Autodesk Inventor part; units mm, degrees
(part 2 of 3)
  line L954 (9.5722, 12.2732) -> (9.481, 12.2224)
  line L955 (9.481, 12.2224) -> (9.3887, 12.173)
  line L956 (9.3887, 12.173) -> (9.2008, 12.0779)
  line L957 (9.2008, 12.0779) -> (8.8135, 11.9014)
  line L958 (8.8135, 11.9014) -> (8.4127, 11.7415)
  line L959 (8.4127, 11.7415) -> (7.9999, 11.5967)
  line L960 (7.9999, 11.5967) -> (7.5762, 11.4663)
  line L961 (7.5762, 11.4663) -> (7.1423, 11.3497)
  line L962 (7.1423, 11.3497) -> (6.777, 11.8009)
  line L963 (6.777, 11.8009) -> (6.9813, 12.201)
  line L964 (6.9813, 12.201) -> (7.1969, 12.5884)
  line L965 (7.1969, 12.5884) -> (7.4243, 12.9621)
  line L966 (7.4243, 12.9621) -> (7.6641, 13.3208)
  line L967 (7.6641, 13.3208) -> (7.9172, 13.663)
  line L968 (7.9172, 13.663) -> (8.0493, 13.827)
  line L969 (8.0493, 13.827) -> (8.1169, 13.907)
  line L970 (8.1169, 13.907) -> (8.1855, 13.9856)
  line L971 (8.1855, 13.9856) -> (7.7098, 14.6404)
  line L972 (7.7098, 14.6404) -> (7.6138, 14.5994)
  line L973 (7.6138, 14.5994) -> (7.5168, 14.5599)
  line L974 (7.5168, 14.5599) -> (7.32, 14.4849)
  line L975 (7.32, 14.4849) -> (6.9164, 14.3499)
  line L976 (6.9164, 14.3499) -> (6.5011, 14.2327)
  line L977 (6.5011, 14.2327) -> (6.0755, 14.1319)
  line L978 (6.0755, 14.1319) -> (5.6404, 14.0465)
  line L979 (5.6404, 14.0465) -> (5.1967, 13.9759)
  line L980 (5.1967, 13.9759) -> (4.8805, 14.4628)
  line L981 (4.8805, 14.4628) -> (5.1255, 14.8394)
  line L982 (5.1255, 14.8394) -> (5.3805, 15.2021)
  line L983 (5.3805, 15.2021) -> (5.6457, 15.55)
  line L984 (5.6457, 15.55) -> (5.9217, 15.8817)
  line L985 (5.9217, 15.8817) -> (6.2092, 16.1955)
  line L986 (6.2092, 16.1955) -> (6.3577, 16.3448)
  line L987 (6.3577, 16.3448) -> (6.4333, 16.4173)
  line L988 (6.4333, 16.4173) -> (6.5097, 16.4883)
  line L989 (6.5097, 16.4883) -> (6.1051, 17.1892)
  line L990 (6.1051, 17.1892) -> (6.0053, 17.1585)
  line L991 (6.0053, 17.1585) -> (5.9047, 17.1293)
  line L992 (5.9047, 17.1293) -> (5.7012, 17.0754)
  line L993 (5.7012, 17.0754) -> (5.2857, 16.9833)
  line L994 (5.2857, 16.9833) -> (4.8604, 16.9101)
  line L995 (4.8604, 16.9101) -> (4.4265, 16.8544)
  line L996 (4.4265, 16.8544) -> (3.9849, 16.8149)
  line L997 (3.9849, 16.8149) -> (3.5363, 16.7911)
  line L998 (3.5363, 16.7911) -> (3.2727, 17.3084)
  line L999 (3.2727, 17.3084) -> (3.5558, 17.6573)
  line L1000 (3.5558, 17.6573) -> (3.8472, 17.9913)
  line L1001 (3.8472, 17.9913) -> (4.1474, 18.3096)
  line L1002 (4.1474, 18.3096) -> (4.4565, 18.6106)
  line L1003 (4.4565, 18.6106) -> (4.7752, 18.8927)
  line L1004 (4.7752, 18.8927) -> (4.9385, 19.0256)
  line L1005 (4.9385, 19.0256) -> (5.0212, 19.0899)
  line L1006 (5.0212, 19.0899) -> (5.1047, 19.1525)
  line L1007 (5.1047, 19.1525) -> (4.7756, 19.8919)
  line L1008 (4.7756, 19.8919) -> (4.6731, 19.8717)
  line L1009 (4.6731, 19.8717) -> (4.5701, 19.8532)
  line L1010 (4.5701, 19.8532) -> (4.362, 19.8208)
  line L1011 (4.362, 19.8208) -> (3.9391, 19.7727)
  line L1012 (3.9391, 19.7727) -> (3.5085, 19.7444)
  line L1013 (3.5085, 19.7444) -> (3.0712, 19.7343)
  line L1014 (3.0712, 19.7343) -> (2.6279, 19.7412)
  line L1015 (2.6279, 19.7412) -> (2.1792, 19.7644)
  line L1016 (2.1792, 19.7644) -> (1.9712, 20.3064)
  line L1017 (1.9712, 20.3064) -> (2.2891, 20.6238)
  line L1018 (2.2891, 20.6238) -> (2.6139, 20.9256)
  line L1019 (2.6139, 20.9256) -> (2.9457, 21.2107)
  line L1020 (2.9457, 21.2107) -> (3.2846, 21.4778)
  line L1021 (3.2846, 21.4778) -> (3.631, 21.725)
  line L1022 (3.631, 21.725) -> (3.8074, 21.8401)
  line L1023 (3.8074, 21.8401) -> (3.8963, 21.8954)
  line L1024 (3.8963, 21.8954) -> (3.9859, 21.949)
  line L1025 (3.9859, 21.949) -> (3.7358, 22.7186)
  line L1026 (3.7358, 22.7186) -> (3.6319, 22.7093)
  line L1027 (3.6319, 22.7093) -> (3.5274, 22.7017)
  line L1028 (3.5274, 22.7017) -> (3.3171, 22.6913)
  line L1029 (3.3171, 22.6913) -> (2.8915, 22.6876)
  line L1030 (2.8915, 22.6876) -> (2.4603, 22.7045)
  line L1031 (2.4603, 22.7045) -> (2.0243, 22.7401)
  line L1032 (2.0243, 22.7401) -> (1.5842, 22.7933)
  line L1033 (1.5842, 22.7933) -> (1.1404, 22.8633)
  line L1034 (1.1404, 22.8633) -> (0.9901, 23.4241)
  line L1035 (0.9901, 23.4241) -> (1.3395, 23.7065)
  line L1036 (1.3395, 23.7065) -> (1.6941, 23.9727)
  line L1037 (1.6941, 23.9727) -> (2.0538, 24.2216)
  line L1038 (2.0538, 24.2216) -> (2.4188, 24.4518)
  line L1039 (2.4188, 24.4518) -> (2.7892, 24.6613)
  line L1040 (2.7892, 24.6613) -> (2.9766, 24.7575)
  line L1041 (2.9766, 24.7575) -> (3.0708, 24.8031)
  line L1042 (3.0708, 24.8031) -> (3.1655, 24.847)
  line L1043 (3.1655, 24.847) -> (2.9973, 25.6386)
  line L1044 (2.9973, 25.6386) -> (2.8929, 25.6402)
  line L1045 (2.8929, 25.6402) -> (2.7882, 25.6436)
  line L1046 (2.7882, 25.6436) -> (2.5779, 25.6552)
  line L1047 (2.5779, 25.6552) -> (2.1543, 25.696)
  line L1048 (2.1543, 25.696) -> (1.7273, 25.7578)
  line L1049 (1.7273, 25.7578) -> (1.2974, 25.8389)
  line L1050 (1.2974, 25.8389) -> (0.8652, 25.9378)
  line L1051 (0.8652, 25.9378) -> (0.4312, 26.0538)
  line L1052 (0.4312, 26.0538) -> (0.3404, 26.6272)
  line L1053 (0.3404, 26.6272) -> (0.7173, 26.8716)
  line L1054 (0.7173, 26.8716) -> (1.0978, 27.0992)
  line L1055 (1.0978, 27.0992) -> (1.4816, 27.3091)
  line L1056 (1.4816, 27.3091) -> (1.8686, 27.4999)
  line L1057 (1.8686, 27.4999) -> (2.2589, 27.6697)
  line L1058 (2.2589, 27.6697) -> (2.4553, 27.7456)
  line L1059 (2.4553, 27.7456) -> (2.5538, 27.7812)
  line L1060 (2.5538, 27.7812) -> (2.6526, 27.8149)
  line L1061 (2.6526, 27.8149) -> (2.568, 28.6198)
  line L1062 (2.568, 28.6198) -> (2.4644, 28.6323)
  line L1063 (2.4644, 28.6323) -> (2.3606, 28.6466)
  line L1064 (2.3606, 28.6466) -> (2.1527, 28.6801)
  line L1065 (2.1527, 28.6801) -> (1.7356, 28.765)
  line L1066 (1.7356, 28.765) -> (1.3174, 28.8711)
  line L1067 (1.3174, 28.8711) -> (0.8983, 28.9967)
  line L1068 (0.8983, 28.9967) -> (0.4789, 29.1403)
  line L1069 (0.4789, 29.1403) -> (0.0593, 29.3009)
  line L1070 (0.0593, 29.3009) -> (0.029, 29.8807)
  line L1071 (0.029, 29.8807) -> (0.4294, 30.0843)
  line L1072 (0.4294, 30.0843) -> (0.8316, 30.2709)
  line L1073 (0.8316, 30.2709) -> (1.2352, 30.4396)
  line L1074 (1.2352, 30.4396) -> (1.64, 30.5889)
  line L1075 (1.64, 30.5889) -> (2.0459, 30.7169)
  line L1076 (2.0459, 30.7169) -> (2.2492, 30.772)
  line L1077 (2.2492, 30.772) -> (2.3509, 30.797)
  line L1078 (2.3509, 30.797) -> (2.4527, 30.8203)
  line L1079 (2.4527, 30.8203) -> (2.4527, 31.6296)
  circle A0 centre (31.2249, 31.2249) radius 0.5
  line L1080 (62.4057, 32.859) -> (0.0441, 29.5908) construction
derived "Base_part.ipt"
derived "gear_central_part_30.ipt"
sketch "Sketch9" plane through (0, 0, 0) normal (0, 1, 0) x (-1, 0, 0)
  circle A0 centre (0, 0) radius 15
  arc A1 (4.5, -13.2571) -> (5.5, -12.8744) centre (0, 0) ccw
  line L0 (0, 0) -> (20.2233, 0) construction
  line L1 (0, 0) -> (0, -27.3647) construction
  line L2 (0.2121, 2.4395) -> (2.4395, 0.2121)
  line L3 (2.4395, -0.2121) -> (0.2121, -2.4395)
  line L4 (-0.2121, -2.4395) -> (-2.4395, -0.2121)
  line L5 (-2.4395, 0.2121) -> (-0.2121, 2.4395)
  line L6 (0, 2.6517) -> (0, -2.6517) construction
  line L7 (2.6517, 0) -> (-2.6517, 0) construction
  arc A2 (2.4395, -0.2121) -> (2.4395, 0.2121) centre (2.2274, 0) ccw
  arc A3 (-0.2121, -2.4395) -> (0.2121, -2.4395) centre (0, -2.2274) ccw
  arc A4 (-2.4395, 0.2121) -> (-2.4395, -0.2121) centre (-2.2274, 0) ccw
  arc A5 (0.2121, 2.4395) -> (-0.2121, 2.4395) centre (0, 2.2274) ccw
  line L8 (-3.1466, -0.9192) -> (-0.9192, -3.1466)
  arc A6 (-0.9192, -3.1466) -> (0.9192, -3.1466) centre (0, -2.2274) ccw
  line L9 (0.9192, -3.1466) -> (3.1466, -0.9192)
  arc A7 (3.1466, -0.9192) -> (3.1466, 0.9192) centre (2.2274, 0) ccw
  line L10 (3.1466, 0.9192) -> (0.9192, 3.1466)
  arc A8 (0.9192, 3.1466) -> (-0.9192, 3.1466) centre (0, 2.2274) ccw
  line L11 (-0.9192, 3.1466) -> (-3.1466, 0.9192)
  arc A9 (-3.1466, 0.9192) -> (-3.1466, -0.9192) centre (-2.2274, 0) ccw
  circle A10 centre (10, 0) radius 2.5
  arc A11 (13.4641, -0.5) -> (9.5, -3.4641) centre (10, 0) ccw
  line L12 (3.4274, -0.5) -> (6.5359, -0.5)
  line L13 (3.4274, 0.5) -> (6.5359, 0.5)
  line L14 (13.9911, 0.5) -> (13.4641, 0.5)
  line L15 (13.9911, -0.5) -> (13.4641, -0.5)
  line L16 (0, -5) -> (13.0767, -5) construction
  line L17 (0, -4.5) -> (13.2571, -4.5)
  line L18 (0, -5.5) -> (12.8744, -5.5)
  line L19 (5, 0) -> (5, -13.0767) construction
  line L20 (5.5, 12.8744) -> (5.5, -12.8744)
  line L21 (4.5, 13.2571) -> (4.5, -13.2571)
  arc A12 (0, -14) -> (4.5, -13.2571) centre (0, 0) ccw
  arc A13 (5.5, -12.8744) -> (12.8744, -5.5) centre (0, 0) ccw
  arc A14 (12.8744, -5.5) -> (13.2571, -4.5) centre (0, 0) ccw
  arc A15 (13.2571, -4.5) -> (13.9911, -0.5) centre (0, 0) ccw
  arc A16 (13.9911, -0.5) -> (13.9911, 0.5) centre (0, 0) ccw
  arc A17 (13.9911, 0.5) -> (5.5, 12.8744) centre (0, 0) ccw
  line L22 (0.5, -4.5) -> (0.5, -5.5)
  line L23 (10, 0) -> (10, -4.5) construction
  line L24 (10.5, -3.4641) -> (10.5, -4.5)
  line L25 (9.5, -3.4641) -> (9.5, -4.5)
  arc A18 (10.5, -3.4641) -> (13.4641, -0.5) centre (10, 0) ccw
  arc A19 (9.5, -3.4641) -> (10.5, -3.4641) centre (10, 0) ccw
  arc A20 (10.5, 3.4641) -> (9.5, 3.4641) centre (10, 0) ccw
  line L26 (0, -4.5) -> (0, -5.5)
  arc A21 (4.5, 13.2571) -> (0, -14) centre (0, 0) ccw
  arc A22 (5.5, 12.8744) -> (4.5, 13.2571) centre (0, 0) ccw
  line L27 (0, 4.5) -> (0, 5.5)
  line L28 (9.5, 3.4641) -> (9.5, 4.5)
  arc A23 (10.5, 3.4641) -> (9.5, 3.4641) centre (10, 0) ccw
  line L29 (0.5, 4.5) -> (0.5, 5.5)
  line L30 (0, 4.5) -> (13.2571, 4.5)
  line L31 (0, 5) -> (13.0767, 5) construction
  line L32 (0, 5.5) -> (12.8744, 5.5)
  arc A24 (13.2571, 4.5) -> (12.8744, 5.5) centre (0, 0) ccw
  line L33 (10.5, 3.4641) -> (10.5, 4.5)
  arc A25 (2.4395, -0.2121) -> (2.4395, 0.2121) centre (2.2274, 0) ccw
  line L34 (0.2121, 2.4395) -> (2.4395, 0.2121)
  line L35 (0.9192, -3.1466) -> (3.1466, -0.9192)
  arc A26 (0.2121, 2.4395) -> (-0.2121, 2.4395) centre (0, 2.2274) ccw
  line L36 (2.4395, -0.2121) -> (0.2121, -2.4395)
  line L37 (0, 2.6517) -> (0, -2.6517) construction
  line L38 (-2.4395, 0.2121) -> (-0.2121, 2.4395)
  line L39 (-2.6517, 0) -> (2.6517, 0) construction
  arc A27 (-0.2121, -2.4395) -> (0.2121, -2.4395) centre (0, -2.2274) ccw
  line L40 (-0.2121, -2.4395) -> (-2.4395, -0.2121)
  arc A28 (3.1466, -0.9192) -> (3.1466, 0.9192) centre (2.2274, 0) ccw
  line L41 (3.1466, 0.9192) -> (0.9192, 3.1466)
  line L42 (4.5, 0.5) -> (5.5, 0.5)
  line L43 (4.5, 0) -> (5.5, 0)
  line L44 (-13.2571, 4.5) -> (13.2571, 4.5)
  line L45 (0, 5) -> (13.0767, 5) construction
  arc A29 (14, 0) -> (13.2571, 4.5) centre (0, 0) ccw
  arc A30 (-0.9192, -3.1466) -> (0.9192, -3.1466) centre (0, -2.2274) ccw
  line L46 (-3.1466, -0.9192) -> (-0.9192, -3.1466)
  arc A31 (-12.8744, 5.5) -> (-13.2571, 4.5) centre (0, 0) ccw
  circle A32 centre (0, 10) radius 2.5
  arc A33 (0.5, 13.4641) -> (3.4641, 9.5) centre (0, 10) ccw
  line L47 (0.5, 3.4274) -> (0.5, 6.5359)
  line L48 (-0.5, 3.4274) -> (-0.5, 6.5359)
  arc A34 (3.4641, 10.5) -> (0.5, 13.4641) centre (0, 10) ccw
  line L49 (0, 10) -> (4.5, 10) construction
  line L50 (0.5, 13.9911) -> (0.5, 13.4641)
  arc A35 (4.5, 13.2571) -> (0.5, 13.9911) centre (0, 0) ccw
  line L51 (-12.8744, 5.5) -> (12.8744, 5.5)
  arc A36 (0.5, 13.9911) -> (-0.5, 13.9911) centre (0, 0) ccw
  line L52 (-0.5, 13.9911) -> (-0.5, 13.4641)
  arc A37 (13.2571, 4.5) -> (12.8744, 5.5) centre (0, 0) ccw
  arc A38 (3.4641, 9.5) -> (3.4641, 10.5) centre (0, 10) ccw
  line L53 (3.4641, 9.5) -> (4.5, 9.5)
  line L54 (3.4641, 10.5) -> (4.5, 10.5)
  arc A39 (5.5, 12.8744) -> (4.5, 13.2571) centre (0, 0) ccw
  line L55 (4.5, 0) -> (4.5, 13.2571)
  line L56 (5, 0) -> (5, 13.0767) construction
  line L57 (5.5, 0) -> (5.5, 12.8744)
  arc A40 (12.8744, 5.5) -> (5.5, 12.8744) centre (0, 0) ccw
  line L58 (-0.9192, 3.1466) -> (-3.1466, 0.9192)
  arc A41 (-3.4641, 10.5) -> (-3.4641, 9.5) centre (0, 10) ccw
  arc A42 (-3.4641, 10.5) -> (-3.4641, 9.5) centre (0, 10) ccw
  line L59 (-3.4641, 10.5) -> (-4.5, 10.5)
  line L60 (-4.5, 0) -> (-4.5, 13.2571)
  line L61 (-5, 0) -> (-5, 13.0767) construction
  line L62 (-5.5, 0) -> (-5.5, 12.8744)
  arc A43 (-4.5, 13.2571) -> (-5.5, 12.8744) centre (0, 0) ccw
  arc A44 (-0.5, 13.9911) -> (-12.8744, 5.5) centre (0, 0) ccw
  line L63 (-3.4641, 9.5) -> (-4.5, 9.5)
  line L64 (-4.5, 0.5) -> (-5.5, 0.5)
  line L65 (-4.5, 0) -> (-5.5, 0)
  arc A45 (-2.4395, 0.2121) -> (-2.4395, -0.2121) centre (-2.2274, 0) ccw
  arc A46 (-3.1466, 0.9192) -> (-3.1466, -0.9192) centre (-2.2274, 0) ccw
  arc A47 (0.9192, 3.1466) -> (-0.9192, 3.1466) centre (0, 2.2274) ccw
  arc A48 (0.2121, 2.4395) -> (-0.2121, 2.4395) centre (0, 2.2274) ccw
  line L66 (-2.4395, 0.2121) -> (-0.2121, 2.4395)
  line L67 (3.1466, 0.9192) -> (0.9192, 3.1466)
  arc A49 (-2.4395, 0.2121) -> (-2.4395, -0.2121) centre (-2.2274, 0) ccw
  line L68 (0.2121, 2.4395) -> (2.4395, 0.2121)
  line L69 (-2.6517, 0) -> (2.6517, 0) construction
  line L70 (-0.2121, -2.4395) -> (-2.4395, -0.2121)
  line L71 (0, -2.6517) -> (0, 2.6517) construction
  arc A50 (2.4395, -0.2121) -> (2.4395, 0.2121) centre (2.2274, 0) ccw
  line L72 (2.4395, -0.2121) -> (0.2121, -2.4395)
  arc A51 (0.9192, 3.1466) -> (-0.9192, 3.1466) centre (0, 2.2274) ccw
  line L73 (-0.9192, 3.1466) -> (-3.1466, 0.9192)
  line L74 (-0.5, 4.5) -> (-0.5, 5.5)
  line L75 (0, 4.5) -> (0, 5.5)
  line L76 (-4.5, -13.2571) -> (-4.5, 13.2571)
  line L77 (-5, 0) -> (-5, 13.0767) construction
  arc A52 (0, 14) -> (-4.5, 13.2571) centre (0, 0) ccw
  arc A53 (3.1466, -0.9192) -> (3.1466, 0.9192) centre (2.2274, 0) ccw
  line L78 (0.9192, -3.1466) -> (3.1466, -0.9192)
  arc A54 (-5.5, -12.8744) -> (-4.5, -13.2571) centre (0, 0) ccw
  circle A55 centre (-10, 0) radius 2.5
  arc A56 (-13.4641, 0.5) -> (-9.5, 3.4641) centre (-10, 0) ccw
  line L79 (-3.4274, 0.5) -> (-6.5359, 0.5)
  line L80 (-3.4274, -0.5) -> (-6.5359, -0.5)
  arc A57 (-10.5, 3.4641) -> (-13.4641, 0.5) centre (-10, 0) ccw
  line L81 (-10, 0) -> (-10, 4.5) construction
  line L82 (-13.9911, 0.5) -> (-13.4641, 0.5)
  arc A58 (-13.2571, 4.5) -> (-13.9911, 0.5) centre (0, 0) ccw
  line L83 (-5.5, -12.8744) -> (-5.5, 12.8744)
  arc A59 (-13.9911, 0.5) -> (-13.9911, -0.5) centre (0, 0) ccw
  line L84 (-13.9911, -0.5) -> (-13.4641, -0.5)
  arc A60 (-4.5, 13.2571) -> (-5.5, 12.8744) centre (0, 0) ccw
  arc A61 (-9.5, 3.4641) -> (-10.5, 3.4641) centre (-10, 0) ccw
  line L85 (-9.5, 3.4641) -> (-9.5, 4.5)
  line L86 (-10.5, 3.4641) -> (-10.5, 4.5)
  arc A62 (-12.8744, 5.5) -> (-13.2571, 4.5) centre (0, 0) ccw
  line L87 (0, 4.5) -> (-13.2571, 4.5)
  line L88 (0, 5) -> (-13.0767, 5) construction
  line L89 (0, 5.5) -> (-12.8744, 5.5)
  arc A63 (-5.5, 12.8744) -> (-12.8744, 5.5) centre (0, 0) ccw
  line L90 (-3.1466, -0.9192) -> (-0.9192, -3.1466)
  arc A64 (-10.5, -3.4641) -> (-9.5, -3.4641) centre (-10, 0) ccw
  arc A65 (-10.5, -3.4641) -> (-9.5, -3.4641) centre (-10, 0) ccw
  line L91 (-10.5, -3.4641) -> (-10.5, -4.5)
  line L92 (0, -4.5) -> (-13.2571, -4.5)
  line L93 (0, -5) -> (-13.0767, -5) construction
  line L94 (0, -5.5) -> (-12.8744, -5.5)
  arc A66 (-13.2571, -4.5) -> (-12.8744, -5.5) centre (0, 0) ccw
  arc A67 (-13.9911, -0.5) -> (-5.5, -12.8744) centre (0, 0) ccw
  line L95 (-9.5, -3.4641) -> (-9.5, -4.5)
  line L96 (-0.5, -4.5) -> (-0.5, -5.5)
  line L97 (0, -4.5) -> (0, -5.5)
  arc A68 (-0.2121, -2.4395) -> (0.2121, -2.4395) centre (0, -2.2274) ccw
  arc A69 (-0.9192, -3.1466) -> (0.9192, -3.1466) centre (0, -2.2274) ccw
  arc A70 (-3.1466, 0.9192) -> (-3.1466, -0.9192) centre (-2.2274, 0) ccw
  arc A71 (-2.4395, 0.2121) -> (-2.4395, -0.2121) centre (-2.2274, 0) ccw
  line L98 (-0.2121, -2.4395) -> (-2.4395, -0.2121)
  line L99 (-0.9192, 3.1466) -> (-3.1466, 0.9192)
  arc A72 (-0.2121, -2.4395) -> (0.2121, -2.4395) centre (0, -2.2274) ccw
  line L100 (-2.4395, 0.2121) -> (-0.2121, 2.4395)
  line L101 (0, -2.6517) -> (0, 2.6517) construction
  line L102 (2.4395, -0.2121) -> (0.2121, -2.4395)
  line L103 (2.6517, 0) -> (-2.6517, 0) construction
  arc A73 (0.2121, 2.4395) -> (-0.2121, 2.4395) centre (0, 2.2274) ccw
  line L104 (0.2121, 2.4395) -> (2.4395, 0.2121)
  arc A74 (-3.1466, 0.9192) -> (-3.1466, -0.9192) centre (-2.2274, 0) ccw
  line L105 (-3.1466, -0.9192) -> (-0.9192, -3.1466)
  line L106 (-4.5, -0.5) -> (-5.5, -0.5)
  line L107 (-4.5, 0) -> (-5.5, 0)
  line L108 (13.2571, -4.5) -> (-13.2571, -4.5)
  line L109 (0, -5) -> (-13.0767, -5) construction
  arc A75 (-14, 0) -> (-13.2571, -4.5) centre (0, 0) ccw
  arc A76 (0.9192, 3.1466) -> (-0.9192, 3.1466) centre (0, 2.2274) ccw
  line L110 (3.1466, 0.9192) -> (0.9192, 3.1466)
  arc A77 (12.8744, -5.5) -> (13.2571, -4.5) centre (0, 0) ccw
  circle A78 centre (0, -10) radius 2.5
  arc A79 (-0.5, -13.4641) -> (-3.4641, -9.5) centre (0, -10) ccw
  line L111 (-0.5, -3.4274) -> (-0.5, -6.5359)
  line L112 (0.5, -3.4274) -> (0.5, -6.5359)
  arc A80 (-3.4641, -10.5) -> (-0.5, -13.4641) centre (0, -10) ccw
  line L113 (0, -10) -> (-4.5, -10) construction
  line L114 (-0.5, -13.9911) -> (-0.5, -13.4641)
  arc A81 (-4.5, -13.2571) -> (-0.5, -13.9911) centre (0, 0) ccw
  line L115 (12.8744, -5.5) -> (-12.8744, -5.5)
  arc A82 (-0.5, -13.9911) -> (0.5, -13.9911) centre (0, 0) ccw
  line L116 (0.5, -13.9911) -> (0.5, -13.4641)
  arc A83 (-13.2571, -4.5) -> (-12.8744, -5.5) centre (0, 0) ccw
  arc A84 (-3.4641, -9.5) -> (-3.4641, -10.5) centre (0, -10) ccw
  line L117 (-3.4641, -9.5) -> (-4.5, -9.5)
  line L118 (-3.4641, -10.5) -> (-4.5, -10.5)
  arc A85 (-5.5, -12.8744) -> (-4.5, -13.2571) centre (0, 0) ccw
  line L119 (-4.5, 0) -> (-4.5, -13.2571)
  line L120 (-5, 0) -> (-5, -13.0767) construction
  line L121 (-5.5, 0) -> (-5.5, -12.8744)
  arc A86 (-12.8744, -5.5) -> (-5.5, -12.8744) centre (0, 0) ccw
  line L122 (0.9192, -3.1466) -> (3.1466, -0.9192)
  arc A87 (3.4641, -10.5) -> (3.4641, -9.5) centre (0, -10) ccw
  arc A88 (3.4641, -10.5) -> (3.4641, -9.5) centre (0, -10) ccw
  line L123 (3.4641, -10.5) -> (4.5, -10.5)
  line L124 (4.5, 0) -> (4.5, -13.2571)
  line L125 (5, 0) -> (5, -13.0767) construction
  line L126 (5.5, 0) -> (5.5, -12.8744)
  arc A89 (4.5, -13.2571) -> (5.5, -12.8744) centre (0, 0) ccw
  arc A90 (0.5, -13.9911) -> (12.8744, -5.5) centre (0, 0) ccw
  line L127 (3.4641, -9.5) -> (4.5, -9.5)
  line L128 (4.5, -0.5) -> (5.5, -0.5)
  line L129 (4.5, 0) -> (5.5, 0)
  arc A91 (2.4395, -0.2121) -> (2.4395, 0.2121) centre (2.2274, 0) ccw
  arc A92 (3.1466, -0.9192) -> (3.1466, 0.9192) centre (2.2274, 0) ccw
  arc A93 (-0.9192, -3.1466) -> (0.9192, -3.1466) centre (0, -2.2274) ccw
  point P0 (0, 2.2274)
  point P1 (10, 4.5)
  point P2 (-4.5, 10)
  point P3 (-2.2274, 0)
  point P4 (-10, -4.5)
  point P5 (0, -2.2274)
  point P6 (4.5, -10)
  point P7 (2.2274, 0)
sketch "Sketch7" plane through (0, 0, 0) normal (0, 1, 0) x (-1, 0, 0)
  line L0 (0, 31.2236) -> (0, -31.2236) construction
  arc A0 (4.5, 27.4052) -> (-4.5, 27.4052) centre (0, 0) ccw
  line L1 (5.5, 13.9553) -> (5.5, 27.2222)
  line L2 (4.5, 14.3091) -> (4.5, 27.4052)
  line L3 (5.5, 0) -> (5.5, 12.8744) projected
  line L4 (4.5, 0) -> (4.5, 13.2571) projected
  line L5 (-4.5, 0) -> (-4.5, 13.2571) projected
  line L6 (-5.5, -12.8744) -> (-5.5, 12.8744) projected
  circle A1 centre (0, 0) radius 15 projected
  line L7 (-4.5, 14.3091) -> (-4.5, 27.4052)
  line L8 (-5.5, 13.9553) -> (-5.5, 27.2222)
  arc A2 (5.5, 27.2222) -> (4.5, 27.4052) centre (0, 0) ccw
  arc A3 (-5.5, 27.2222) -> (5.5, 27.2222) centre (0, 0) ccw
  arc A4 (-4.5, 27.4052) -> (-5.5, 27.2222) centre (0, 0) ccw
  arc A5 (5.5, 13.9553) -> (4.5, 14.3091) centre (0, 0) ccw
  arc A6 (-4.5, 14.3091) -> (-5.5, 13.9553) centre (0, 0) ccw
  arc A7 (-14.3091, -4.5) -> (-13.9553, -5.5) centre (0, 0) ccw
  arc A8 (-13.9553, 5.5) -> (-14.3091, 4.5) centre (0, 0) ccw
  line L9 (-13.9553, 5.5) -> (-27.2222, 5.5)
  line L10 (-14.3091, 4.5) -> (-27.4052, 4.5)
  arc A9 (-27.2222, 5.5) -> (-27.4052, 4.5) centre (0, 0) ccw
  line L11 (-14.3091, -4.5) -> (-27.4052, -4.5)
  line L12 (-13.9553, -5.5) -> (-27.2222, -5.5)
  arc A10 (-27.4052, -4.5) -> (-27.2222, -5.5) centre (0, 0) ccw
  arc A11 (4.5, -14.3091) -> (5.5, -13.9553) centre (0, 0) ccw
  arc A12 (-5.5, -13.9553) -> (-4.5, -14.3091) centre (0, 0) ccw
  line L13 (-5.5, -13.9553) -> (-5.5, -27.2222)
  line L14 (-4.5, -14.3091) -> (-4.5, -27.4052)
  arc A13 (-5.5, -27.2222) -> (-4.5, -27.4052) centre (0, 0) ccw
  line L15 (4.5, -14.3091) -> (4.5, -27.4052)
  line L16 (5.5, -13.9553) -> (5.5, -27.2222)
  arc A14 (4.5, -27.4052) -> (5.5, -27.2222) centre (0, 0) ccw
  arc A15 (14.3091, 4.5) -> (13.9553, 5.5) centre (0, 0) ccw
  arc A16 (13.9553, -5.5) -> (14.3091, -4.5) centre (0, 0) ccw
  line L17 (13.9553, -5.5) -> (27.2222, -5.5)
  line L18 (14.3091, -4.5) -> (27.4052, -4.5)
  arc A17 (27.2222, -5.5) -> (27.4052, -4.5) centre (0, 0) ccw
  line L19 (14.3091, 4.5) -> (27.4052, 4.5)
  line L20 (13.9553, 5.5) -> (27.2222, 5.5)
  arc A18 (27.4052, 4.5) -> (27.2222, 5.5) centre (0, 0) ccw
  arc A19 (14.7224, 8.5) -> (8.5, 14.7224) centre (0, 0) ccw
  line L21 (16.4545, 7.5) -> (21.7915, 7.5)
  line L22 (7.5, 16.4545) -> (7.5, 21.7915)
  arc A20 (23.6249, 10.2993) -> (10.2993, 23.6249) centre (0, 0) ccw
  arc A21 (21.7915, 7.5) -> (23.6249, 10.2993) centre (21.7915, 9.5) ccw
  arc A22 (14.7224, 8.5) -> (16.4545, 7.5) centre (16.4545, 9.5) ccw
  arc A23 (7.5, 16.4545) -> (8.5, 14.7224) centre (9.5, 16.4545) ccw
  arc A24 (10.2993, 23.6249) -> (7.5, 21.7915) centre (9.5, 21.7915) ccw
  arc A25 (-16.4545, 7.5) -> (-14.7224, 8.5) centre (-16.4545, 9.5) ccw
  line L23 (-16.4545, 7.5) -> (-21.7915, 7.5)
  arc A26 (-23.6249, 10.2993) -> (-21.7915, 7.5) centre (-21.7915, 9.5) ccw
  arc A27 (-8.5, 14.7224) -> (-14.7224, 8.5) centre (0, 0) ccw
  arc A28 (-10.2993, 23.6249) -> (-23.6249, 10.2993) centre (0, 0) ccw
  arc A29 (-8.5, 14.7224) -> (-7.5, 16.4545) centre (-9.5, 16.4545) ccw
  line L24 (-7.5, 16.4545) -> (-7.5, 21.7915)
  arc A30 (-7.5, 21.7915) -> (-10.2993, 23.6249) centre (-9.5, 21.7915) ccw
  arc A31 (-7.5, -16.4545) -> (-8.5, -14.7224) centre (-9.5, -16.4545) ccw
  line L25 (-7.5, -16.4545) -> (-7.5, -21.7915)
  arc A32 (-10.2993, -23.6249) -> (-7.5, -21.7915) centre (-9.5, -21.7915) ccw
  arc A33 (-14.7224, -8.5) -> (-8.5, -14.7224) centre (0, 0) ccw
  arc A34 (-23.6249, -10.2993) -> (-10.2993, -23.6249) centre (0, 0) ccw
  arc A35 (-14.7224, -8.5) -> (-16.4545, -7.5) centre (-16.4545, -9.5) ccw
  line L26 (-16.4545, -7.5) -> (-21.7915, -7.5)
  arc A36 (-21.7915, -7.5) -> (-23.6249, -10.2993) centre (-21.7915, -9.5) ccw
  arc A37 (16.4545, -7.5) -> (14.7224, -8.5) centre (16.4545, -9.5) ccw
  line L27 (16.4545, -7.5) -> (21.7915, -7.5)
  arc A38 (23.6249, -10.2993) -> (21.7915, -7.5) centre (21.7915, -9.5) ccw
  arc A39 (8.5, -14.7224) -> (14.7224, -8.5) centre (0, 0) ccw
  arc A40 (10.2993, -23.6249) -> (23.6249, -10.2993) centre (0, 0) ccw
  arc A41 (8.5, -14.7224) -> (7.5, -16.4545) centre (9.5, -16.4545) ccw
  line L28 (7.5, -16.4545) -> (7.5, -21.7915)
  arc A42 (7.5, -21.7915) -> (10.2993, -23.6249) centre (9.5, -21.7915) ccw
  line L29 (-28.7116, 1.9099) -> (-28.812, 1.9385)
  line L30 (-28.812, 1.9385) -> (-28.9123, 1.9688)
  line L31 (-28.9123, 1.9688) -> (-29.1124, 2.0344)
  line L32 (-29.1124, 2.0344) -> (-29.511, 2.1835)
  line L33 (-29.511, 2.1835) -> (-29.9075, 2.3538)
  line L34 (-29.9075, 2.3538) -> (-30.3018, 2.5433)
  line L35 (-30.3018, 2.5433) -> (-30.6936, 2.7507)
  line L36 (-30.6936, 2.7507) -> (-31.0829, 2.9751)
  line L37 (-31.0829, 2.9751) -> (-31.0222, 3.5524)
  line L38 (-31.0222, 3.5524) -> (-30.5948, 3.6909)
  line L39 (-30.5948, 3.6909) -> (-30.1684, 3.8124)
  line L40 (-30.1684, 3.8124) -> (-29.7433, 3.9158)
  line L41 (-29.7433, 3.9158) -> (-29.3201, 3.9999)
  line L42 (-29.3201, 3.9999) -> (-28.8992, 4.0628)
  line L43 (-28.8992, 4.0628) -> (-28.6898, 4.0854)
  line L44 (-28.6898, 4.0854) -> (-28.5855, 4.0942)
  line L45 (-28.5855, 4.0942) -> (-28.4813, 4.1013)
  line L46 (-28.4813, 4.1013) -> (-28.3547, 4.9006)
  line L47 (-28.3547, 4.9006) -> (-28.4516, 4.9395)
  line L48 (-28.4516, 4.9395) -> (-28.5481, 4.9802)
  line L49 (-28.5481, 4.9802) -> (-28.7403, 5.0664)
  line L50 (-28.7403, 5.0664) -> (-29.1211, 5.2563)
  line L51 (-29.1211, 5.2563) -> (-29.4976, 5.4671)
  line L52 (-29.4976, 5.4671) -> (-29.8699, 5.6968)
  line L53 (-29.8699, 5.6968) -> (-30.2379, 5.944)
  line L54 (-30.2379, 5.944) -> (-30.6016, 6.2078)
  line L55 (-30.6016, 6.2078) -> (-30.4809, 6.7757)
  line L56 (-30.4809, 6.7757) -> (-30.0414, 6.8687)
  line L57 (-30.0414, 6.8687) -> (-29.6046, 6.9449)
  line L58 (-29.6046, 6.9449) -> (-29.1711, 7.0034)
  line L59 (-29.1711, 7.0034) -> (-28.7414, 7.0428)
  line L60 (-28.7414, 7.0428) -> (-28.3162, 7.0614)
  line L61 (-28.3162, 7.0614) -> (-28.1056, 7.0619)
  line L62 (-28.1056, 7.0619) -> (-28.0009, 7.0598)
  line L63 (-28.0009, 7.0598) -> (-27.8966, 7.0559)
  line L64 (-27.8966, 7.0559) -> (-27.6871, 7.8377)
  line L65 (-27.6871, 7.8377) -> (-27.7794, 7.8865)
  line L66 (-27.7794, 7.8865) -> (-27.8711, 7.937)
  line L67 (-27.8711, 7.937) -> (-28.0532, 8.0428)
  line L68 (-28.0532, 8.0428) -> (-28.4122, 8.2714)
  line L69 (-28.4122, 8.2714) -> (-28.7646, 8.5205)
  line L70 (-28.7646, 8.5205) -> (-29.1108, 8.7878)
  line L71 (-29.1108, 8.7878) -> (-29.4509, 9.0722)
  line L72 (-29.4509, 9.0722) -> (-29.7851, 9.3725)
  line L73 (-29.7851, 9.3725) -> (-29.6057, 9.9247)
  line L74 (-29.6057, 9.9247) -> (-29.1588, 9.9713)
  line L75 (-29.1588, 9.9713) -> (-28.7165, 10.0014)
  line L76 (-28.7165, 10.0014) -> (-28.2792, 10.0142)
  line L77 (-28.2792, 10.0142) -> (-27.8478, 10.0085)
  line L78 (-27.8478, 10.0085) -> (-27.423, 9.9825)
  line L79 (-27.423, 9.9825) -> (-27.2135, 9.9611)
  line L80 (-27.2135, 9.9611) -> (-27.1096, 9.948)
  line L81 (-27.1096, 9.948) -> (-27.0062, 9.9333)
  line L82 (-27.0062, 9.9333) -> (-26.7162, 10.6888)
  line L83 (-26.7162, 10.6888) -> (-26.8028, 10.747)
  line L84 (-26.8028, 10.747) -> (-26.8888, 10.8068)
  line L85 (-26.8888, 10.8068) -> (-27.0589, 10.9311)
  line L86 (-27.0589, 10.9311) -> (-27.3919, 11.196)
  line L87 (-27.3919, 11.196) -> (-27.7164, 11.4805)
  line L88 (-27.7164, 11.4805) -> (-28.0328, 11.7826)
  line L89 (-28.0328, 11.7826) -> (-28.3413, 12.1009)
  line L90 (-28.3413, 12.1009) -> (-28.6422, 12.4346)
  line L91 (-28.6422, 12.4346) -> (-28.4061, 12.965)
  line L92 (-28.4061, 12.965) -> (-27.9568, 12.9646)
  line L93 (-27.9568, 12.9646) -> (-27.5138, 12.9483)
  line L94 (-27.5138, 12.9483) -> (-27.0776, 12.9153)
  line L95 (-27.0776, 12.9153) -> (-26.649, 12.8646)
  line L96 (-26.649, 12.8646) -> (-26.2293, 12.7943)
  line L97 (-26.2293, 12.7943) -> (-26.0232, 12.7511)
  line L98 (-26.0232, 12.7511) -> (-25.9212, 12.7272)
  line L99 (-25.9212, 12.7272) -> (-25.82, 12.7018)
  line L100 (-25.82, 12.7018) -> (-25.4526, 13.4229)
  line L101 (-25.4526, 13.4229) -> (-25.5327, 13.4898)
  line L102 (-25.5327, 13.4898) -> (-25.6119, 13.5583)
  line L103 (-25.6119, 13.5583) -> (-25.768, 13.6996)
  line L104 (-25.768, 13.6996) -> (-26.0716, 13.9979)
  line L105 (-26.0716, 13.9979) -> (-26.3645, 14.3148)
  line L106 (-26.3645, 14.3148) -> (-26.6476, 14.6483)
  line L107 (-26.6476, 14.6483) -> (-26.9212, 14.9971)
  line L108 (-26.9212, 14.9971) -> (-27.1855, 15.3604)
  line L109 (-27.1855, 15.3604) -> (-26.8953, 15.8632)
  line L110 (-26.8953, 15.8632) -> (-26.4485, 15.8158)
  line L111 (-26.4485, 15.8158) -> (-26.0096, 15.7533)
  line L112 (-26.0096, 15.7533) -> (-25.5792, 15.675)
  line L113 (-25.5792, 15.675) -> (-25.1583, 15.5797)
  line L114 (-25.1583, 15.5797) -> (-24.7482, 15.466)
  line L115 (-24.7482, 15.466) -> (-24.5478, 15.4014)
  line L116 (-24.5478, 15.4014) -> (-24.4488, 15.367)
  line L117 (-24.4488, 15.367) -> (-24.3508, 15.3311)
  line L118 (-24.3508, 15.3311) -> (-23.91, 16.0099)
  line L119 (-23.91, 16.0099) -> (-23.9827, 16.0848)
  line L120 (-23.9827, 16.0848) -> (-24.0544, 16.1612)
  line L121 (-24.0544, 16.1612) -> (-24.1949, 16.3181)
  line L122 (-24.1949, 16.3181) -> (-24.4656, 16.6465)
  line L123 (-24.4656, 16.6465) -> (-24.7238, 16.9922)
  line L124 (-24.7238, 16.9922) -> (-24.9704, 17.3535)
  line L125 (-24.9704, 17.3535) -> (-25.2061, 17.729)
  line L126 (-25.2061, 17.729) -> (-25.431, 18.1179)
  line L127 (-25.431, 18.1179) -> (-25.0898, 18.5876)
  line L128 (-25.0898, 18.5876) -> (-24.6504, 18.4938)
  line L129 (-24.6504, 18.4938) -> (-24.2204, 18.3858)
  line L130 (-24.2204, 18.3858) -> (-23.8006, 18.2628)
  line L131 (-23.8006, 18.2628) -> (-23.392, 18.1241)
  line L132 (-23.392, 18.1241) -> (-22.996, 17.9681)
  line L133 (-22.996, 17.9681) -> (-22.8034, 17.883)
  line L134 (-22.8034, 17.883) -> (-22.7086, 17.8384)
  line L135 (-22.7086, 17.8384) -> (-22.6149, 17.7925)
  line L136 (-22.6149, 17.7925) -> (-22.1056, 18.4214)
  line L137 (-22.1056, 18.4214) -> (-22.17, 18.5036)
  line L138 (-22.17, 18.5036) -> (-22.2333, 18.587)
  line L139 (-22.2333, 18.587) -> (-22.3566, 18.7577)
  line L140 (-22.3566, 18.7577) -> (-22.5915, 19.1126)
  line L141 (-22.5915, 19.1126) -> (-22.8122, 19.4834)
  line L142 (-22.8122, 19.4834) -> (-23.0197, 19.8685)
  line L143 (-23.0197, 19.8685) -> (-23.2148, 20.2666)
  line L144 (-23.2148, 20.2666) -> (-23.3979, 20.6769)
  line L145 (-23.3979, 20.6769) -> (-23.0094, 21.1084)
  line L146 (-23.0094, 21.1084) -> (-22.5822, 20.9692)
  line L147 (-22.5822, 20.9692) -> (-22.1659, 20.8168)
  line L148 (-22.1659, 20.8168) -> (-21.7612, 20.6506)
  line L149 (-21.7612, 20.6506) -> (-21.3694, 20.4699)
  line L150 (-21.3694, 20.4699) -> (-20.9919, 20.2734)
  line L151 (-20.9919, 20.2734) -> (-20.8092, 20.1686)
  line L152 (-20.8092, 20.1686) -> (-20.7196, 20.1144)
  line L153 (-20.7196, 20.1144) -> (-20.6312, 20.0589)
  line L154 (-20.6312, 20.0589) -> (-20.0589, 20.6312)
  line L155 (-20.0589, 20.6312) -> (-20.1144, 20.7196)
  line L156 (-20.1144, 20.7196) -> (-20.1686, 20.8092)
  line L157 (-20.1686, 20.8092) -> (-20.2734, 20.9919)
  line L158 (-20.2734, 20.9919) -> (-20.4699, 21.3694)
  line L159 (-20.4699, 21.3694) -> (-20.6506, 21.7612)
  line L160 (-20.6506, 21.7612) -> (-20.8168, 22.1659)
  line L161 (-20.8168, 22.1659) -> (-20.9692, 22.5822)
  line L162 (-20.9692, 22.5822) -> (-21.1084, 23.0094)
  line L163 (-21.1084, 23.0094) -> (-20.6769, 23.3979)
  line L164 (-20.6769, 23.3979) -> (-20.2666, 23.2148)
  line L165 (-20.2666, 23.2148) -> (-19.8685, 23.0197)
  line L166 (-19.8685, 23.0197) -> (-19.4834, 22.8122)
  line L167 (-19.4834, 22.8122) -> (-19.1126, 22.5915)
  line L168 (-19.1126, 22.5915) -> (-18.7577, 22.3566)
  line L169 (-18.7577, 22.3566) -> (-18.587, 22.2333)
  line L170 (-18.587, 22.2333) -> (-18.5035, 22.17)
  line L171 (-18.5035, 22.17) -> (-18.4214, 22.1056)
  line L172 (-18.4214, 22.1056) -> (-17.7925, 22.6149)
  line L173 (-17.7925, 22.6149) -> (-17.8384, 22.7086)
  line L174 (-17.8384, 22.7086) -> (-17.883, 22.8034)
  line L175 (-17.883, 22.8034) -> (-17.9681, 22.996)
  line L176 (-17.9681, 22.996) -> (-18.1241, 23.392)
  line L177 (-18.1241, 23.392) -> (-18.2628, 23.8006)
  line L178 (-18.2628, 23.8006) -> (-18.3858, 24.2204)
  line L179 (-18.3858, 24.2204) -> (-18.4938, 24.6504)
  line L180 (-18.4938, 24.6504) -> (-18.5876, 25.0898)
  line L181 (-18.5876, 25.0898) -> (-18.1179, 25.431)
  line L182 (-18.1179, 25.431) -> (-17.729, 25.2061)
  line L183 (-17.729, 25.2061) -> (-17.3535, 24.9704)
  line L184 (-17.3535, 24.9704) -> (-16.9922, 24.7238)
  line L185 (-16.9922, 24.7238) -> (-16.6465, 24.4656)
  line L186 (-16.6465, 24.4656) -> (-16.3181, 24.1949)
  line L187 (-16.3181, 24.1949) -> (-16.1612, 24.0544)
  line L188 (-16.1612, 24.0544) -> (-16.0848, 23.9827)
  line L189 (-16.0848, 23.9827) -> (-16.0099, 23.91)
  line L190 (-16.0099, 23.91) -> (-15.3311, 24.3508)
  line L191 (-15.3311, 24.3508) -> (-15.367, 24.4488)
  line L192 (-15.367, 24.4488) -> (-15.4014, 24.5478)
  line L193 (-15.4014, 24.5478) -> (-15.466, 24.7482)
  line L194 (-15.466, 24.7482) -> (-15.5797, 25.1583)
  line L195 (-15.5797, 25.1583) -> (-15.675, 25.5792)
  line L196 (-15.675, 25.5792) -> (-15.7533, 26.0096)
  line L197 (-15.7533, 26.0096) -> (-15.8158, 26.4485)
  line L198 (-15.8158, 26.4485) -> (-15.8632, 26.8952)
  line L199 (-15.8632, 26.8952) -> (-15.3604, 27.1855)
  line L200 (-15.3604, 27.1855) -> (-14.9971, 26.9212)
  line L201 (-14.9971, 26.9212) -> (-14.6483, 26.6476)
  line L202 (-14.6483, 26.6476) -> (-14.3148, 26.3645)
  line L203 (-14.3148, 26.3645) -> (-13.9979, 26.0716)
  line L204 (-13.9979, 26.0716) -> (-13.6996, 25.768)
  line L205 (-13.6996, 25.768) -> (-13.5583, 25.6119)
  line L206 (-13.5583, 25.6119) -> (-13.4898, 25.5327)
  line L207 (-13.4898, 25.5327) -> (-13.4229, 25.4526)
  line L208 (-13.4229, 25.4526) -> (-12.7018, 25.82)
  line L209 (-12.7018, 25.82) -> (-12.7272, 25.9212)
  line L210 (-12.7272, 25.9212) -> (-12.7511, 26.0232)
  line L211 (-12.7511, 26.0232) -> (-12.7943, 26.2293)
  line L212 (-12.7943, 26.2293) -> (-12.8646, 26.649)
  line L213 (-12.8646, 26.649) -> (-12.9153, 27.0776)
  line L214 (-12.9153, 27.0776) -> (-12.9483, 27.5138)
  line L215 (-12.9483, 27.5138) -> (-12.9646, 27.9568)
  line L216 (-12.9646, 27.9568) -> (-12.965, 28.4061)
  line L217 (-12.965, 28.4061) -> (-12.4346, 28.6422)
  line L218 (-12.4346, 28.6422) -> (-12.101, 28.3413)
  line L219 (-12.101, 28.3413) -> (-11.7826, 28.0328)
  line L220 (-11.7826, 28.0328) -> (-11.4805, 27.7164)
  line L221 (-11.4805, 27.7164) -> (-11.196, 27.3919)
  line L222 (-11.196, 27.3919) -> (-10.9311, 27.0589)
  line L223 (-10.9311, 27.0589) -> (-10.8068, 26.8888)
  line L224 (-10.8068, 26.8888) -> (-10.747, 26.8029)
  line L225 (-10.747, 26.8029) -> (-10.6888, 26.7162)
  line L226 (-10.6888, 26.7162) -> (-9.9333, 27.0062)
  line L227 (-9.9333, 27.0062) -> (-9.948, 27.1095)
  line L228 (-9.948, 27.1095) -> (-9.9611, 27.2135)
  line L229 (-9.9611, 27.2135) -> (-9.9825, 27.423)
  line L230 (-9.9825, 27.423) -> (-10.0085, 27.8478)
  line L231 (-10.0085, 27.8478) -> (-10.0142, 28.2792)
  line L232 (-10.0142, 28.2792) -> (-10.0014, 28.7165)
  line L233 (-10.0014, 28.7165) -> (-9.9713, 29.1588)
  line L234 (-9.9713, 29.1588) -> (-9.9247, 29.6057)
  line L235 (-9.9247, 29.6057) -> (-9.3725, 29.7851)
  line L236 (-9.3725, 29.7851) -> (-9.0722, 29.451)
  line L237 (-9.0722, 29.451) -> (-8.7878, 29.1108)
  line L238 (-8.7878, 29.1108) -> (-8.5205, 28.7646)
  line L239 (-8.5205, 28.7646) -> (-8.2715, 28.4122)
  line L240 (-8.2715, 28.4122) -> (-8.0428, 28.0532)
  line L241 (-8.0428, 28.0532) -> (-7.937, 27.8712)
  line L242 (-7.937, 27.8712) -> (-7.8865, 27.7794)
  line L243 (-7.8865, 27.7794) -> (-7.8377, 27.6871)
  line L244 (-7.8377, 27.6871) -> (-7.0559, 27.8966)
  line L245 (-7.0559, 27.8966) -> (-7.0598, 28.0009)
  line L246 (-7.0598, 28.0009) -> (-7.0619, 28.1056)
  line L247 (-7.0619, 28.1056) -> (-7.0614, 28.3162)
  line L248 (-7.0614, 28.3162) -> (-7.0428, 28.7414)
  line L249 (-7.0428, 28.7414) -> (-7.0034, 29.1711)
  line L250 (-7.0034, 29.1711) -> (-6.9449, 29.6046)
  line L251 (-6.9449, 29.6046) -> (-6.8687, 30.0414)
  line L252 (-6.8687, 30.0414) -> (-6.7757, 30.4809)
  line L253 (-6.7757, 30.4809) -> (-6.2078, 30.6016)
  line L254 (-6.2078, 30.6016) -> (-5.944, 30.2379)
  line L255 (-5.944, 30.2379) -> (-5.6968, 29.8699)
  line L256 (-5.6968, 29.8699) -> (-5.4671, 29.4976)
  line L257 (-5.4671, 29.4976) -> (-5.2563, 29.1211)
  line L258 (-5.2563, 29.1211) -> (-5.0664, 28.7403)
  line L259 (-5.0664, 28.7403) -> (-4.9802, 28.5481)
  line L260 (-4.9802, 28.5481) -> (-4.9395, 28.4516)
  line L261 (-4.9395, 28.4516) -> (-4.9006, 28.3547)
  line L262 (-4.9006, 28.3547) -> (-4.1013, 28.4813)
  line L263 (-4.1013, 28.4813) -> (-4.0942, 28.5855)
  line L264 (-4.0942, 28.5855) -> (-4.0854, 28.6898)
  line L265 (-4.0854, 28.6898) -> (-4.0628, 28.8992)
  line L266 (-4.0628, 28.8992) -> (-3.9999, 29.3201)
  line L267 (-3.9999, 29.3201) -> (-3.9158, 29.7433)
  line L268 (-3.9158, 29.7433) -> (-3.8124, 30.1684)
  line L269 (-3.8124, 30.1684) -> (-3.6909, 30.5948)
  line L270 (-3.6909, 30.5948) -> (-3.5525, 31.0222)
  line L271 (-3.5525, 31.0222) -> (-2.9751, 31.0829)
  line L272 (-2.9751, 31.0829) -> (-2.7507, 30.6936)
  line L273 (-2.7507, 30.6936) -> (-2.5433, 30.3018)
  line L274 (-2.5433, 30.3018) -> (-2.3538, 29.9075)
  line L275 (-2.3538, 29.9075) -> (-2.1835, 29.511)
  line L276 (-2.1835, 29.511) -> (-2.0344, 29.1124)
  line L277 (-2.0344, 29.1124) -> (-1.9688, 28.9123)
  line L278 (-1.9688, 28.9123) -> (-1.9385, 28.812)
  line L279 (-1.9385, 28.812) -> (-1.9099, 28.7116)
  line L280 (-1.9099, 28.7116) -> (-1.1017, 28.754)
  line L281 (-1.1017, 28.754) -> (-1.0838, 28.8568)
  line L282 (-1.0838, 28.8568) -> (-1.0641, 28.9597)
  line L283 (-1.0641, 28.9597) -> (-1.0198, 29.1656)
  line L284 (-1.0198, 29.1656) -> (-0.9132, 29.5776)
  line L285 (-0.9132, 29.5776) -> (-0.7853, 29.9897)
  line L286 (-0.7853, 29.9897) -> (-0.638, 30.4016)
  line L287 (-0.638, 30.4016) -> (-0.4727, 30.813)
  line L288 (-0.4727, 30.813) -> (-0.2903, 31.2236)
  line L289 (-0.2903, 31.2236) -> (0.2903, 31.2236)
  line L290 (0.2903, 31.2236) -> (0.4727, 30.813)
  line L291 (0.4727, 30.813) -> (0.638, 30.4016)
  line L292 (0.638, 30.4016) -> (0.7853, 29.9897)
  line L293 (0.7853, 29.9897) -> (0.9132, 29.5776)
  line L294 (0.9132, 29.5776) -> (1.0198, 29.1656)
  line L295 (1.0198, 29.1656) -> (1.0641, 28.9597)
  line L296 (1.0641, 28.9597) -> (1.0838, 28.8568)
  line L297 (1.0838, 28.8568) -> (1.1017, 28.754)
  line L298 (1.1017, 28.754) -> (1.9099, 28.7116)
  line L299 (1.9099, 28.7116) -> (1.9385, 28.812)
  line L300 (1.9385, 28.812) -> (1.9688, 28.9123)
  line L301 (1.9688, 28.9123) -> (2.0344, 29.1124)
  line L302 (2.0344, 29.1124) -> (2.1835, 29.511)
  line L303 (2.1835, 29.511) -> (2.3538, 29.9075)
  line L304 (2.3538, 29.9075) -> (2.5433, 30.3018)
  line L305 (2.5433, 30.3018) -> (2.7507, 30.6936)
  line L306 (2.7507, 30.6936) -> (2.9751, 31.0829)
  line L307 (2.9751, 31.0829) -> (3.5524, 31.0222)
  line L308 (3.5524, 31.0222) -> (3.6909, 30.5948)
  line L309 (3.6909, 30.5948) -> (3.8123, 30.1684)
  line L310 (3.8123, 30.1684) -> (3.9158, 29.7434)
  line L311 (3.9158, 29.7434) -> (3.9999, 29.3201)
  line L312 (3.9999, 29.3201) -> (4.0628, 28.8992)
  line L313 (4.0628, 28.8992) -> (4.0854, 28.6898)
  line L314 (4.0854, 28.6898) -> (4.0942, 28.5855)
  line L315 (4.0942, 28.5855) -> (4.1013, 28.4813)
  line L316 (4.1013, 28.4813) -> (4.9006, 28.3547)
  line L317 (4.9006, 28.3547) -> (4.9395, 28.4516)
  line L318 (4.9395, 28.4516) -> (4.9802, 28.5481)
  line L319 (4.9802, 28.5481) -> (5.0664, 28.7403)
  line L320 (5.0664, 28.7403) -> (5.2563, 29.1211)
  line L321 (5.2563, 29.1211) -> (5.4671, 29.4976)
  line L322 (5.4671, 29.4976) -> (5.6968, 29.8699)
  line L323 (5.6968, 29.8699) -> (5.944, 30.2379)
  line L324 (5.944, 30.2379) -> (6.2078, 30.6016)
  line L325 (6.2078, 30.6016) -> (6.7757, 30.4809)
  line L326 (6.7757, 30.4809) -> (6.8687, 30.0414)
  line L327 (6.8687, 30.0414) -> (6.9449, 29.6046)
  line L328 (6.9449, 29.6046) -> (7.0034, 29.1711)
  line L329 (7.0034, 29.1711) -> (7.0428, 28.7414)
  line L330 (7.0428, 28.7414) -> (7.0614, 28.3162)
  line L331 (7.0614, 28.3162) -> (7.0619, 28.1056)
  line L332 (7.0619, 28.1056) -> (7.0598, 28.0009)
  line L333 (7.0598, 28.0009) -> (7.0559, 27.8966)
  line L334 (7.0559, 27.8966) -> (7.8377, 27.6871)
  line L335 (7.8377, 27.6871) -> (7.8865, 27.7794)
  line L336 (7.8865, 27.7794) -> (7.937, 27.8712)
  line L337 (7.937, 27.8712) -> (8.0428, 28.0532)
  line L338 (8.0428, 28.0532) -> (8.2714, 28.4122)
  line L339 (8.2714, 28.4122) -> (8.5205, 28.7646)
  line L340 (8.5205, 28.7646) -> (8.7878, 29.1108)
  line L341 (8.7878, 29.1108) -> (9.0722, 29.451)
  line L342 (9.0722, 29.451) -> (9.3725, 29.7851)
  line L343 (9.3725, 29.7851) -> (9.9247, 29.6057)
  line L344 (9.9247, 29.6057) -> (9.9713, 29.1588)
  line L345 (9.9713, 29.1588) -> (10.0014, 28.7165)
  line L346 (10.0014, 28.7165) -> (10.0142, 28.2792)
  line L347 (10.0142, 28.2792) -> (10.0085, 27.8478)
  line L348 (10.0085, 27.8478) -> (9.9825, 27.423)
  line L349 (9.9825, 27.423) -> (9.9611, 27.2135)
  line L350 (9.9611, 27.2135) -> (9.948, 27.1095)
  line L351 (9.948, 27.1095) -> (9.9333, 27.0062)
  line L352 (9.9333, 27.0062) -> (10.6888, 26.7162)
  line L353 (10.6888, 26.7162) -> (10.747, 26.8029)
  line L354 (10.747, 26.8029) -> (10.8068, 26.8888)
  line L355 (10.8068, 26.8888) -> (10.9311, 27.0589)
  line L356 (10.9311, 27.0589) -> (11.196, 27.3919)
  line L357 (11.196, 27.3919) -> (11.4805, 27.7164)
  line L358 (11.4805, 27.7164) -> (11.7826, 28.0328)
  line L359 (11.7826, 28.0328) -> (12.1009, 28.3413)
  line L360 (12.1009, 28.3413) -> (12.4346, 28.6422)
  line L361 (12.4346, 28.6422) -> (12.965, 28.4061)
  line L362 (12.965, 28.4061) -> (12.9646, 27.9568)
  line L363 (12.9646, 27.9568) -> (12.9483, 27.5137)
  line L364 (12.9483, 27.5137) -> (12.9153, 27.0776)
  line L365 (12.9153, 27.0776) -> (12.8646, 26.649)
  line L366 (12.8646, 26.649) -> (12.7943, 26.2293)
  line L367 (12.7943, 26.2293) -> (12.7511, 26.0232)
  line L368 (12.7511, 26.0232) -> (12.7272, 25.9212)
  line L369 (12.7272, 25.9212) -> (12.7018, 25.82)
  line L370 (12.7018, 25.82) -> (13.4229, 25.4526)
  line L371 (13.4229, 25.4526) -> (13.4898, 25.5327)
  line L372 (13.4898, 25.5327) -> (13.5583, 25.6119)
  line L373 (13.5583, 25.6119) -> (13.6996, 25.768)
  line L374 (13.6996, 25.768) -> (13.9979, 26.0716)
  line L375 (13.9979, 26.0716) -> (14.3148, 26.3645)
  line L376 (14.3148, 26.3645) -> (14.6483, 26.6476)
  line L377 (14.6483, 26.6476) -> (14.9971, 26.9212)
  line L378 (14.9971, 26.9212) -> (15.3604, 27.1855)
  line L379 (15.3604, 27.1855) -> (15.8632, 26.8952)
  line L380 (15.8632, 26.8952) -> (15.8158, 26.4485)
  line L381 (15.8158, 26.4485) -> (15.7533, 26.0096)
  line L382 (15.7533, 26.0096) -> (15.675, 25.5792)
  line L383 (15.675, 25.5792) -> (15.5797, 25.1583)
  line L384 (15.5797, 25.1583) -> (15.466, 24.7482)
  line L385 (15.466, 24.7482) -> (15.4014, 24.5478)
  line L386 (15.4014, 24.5478) -> (15.367, 24.4488)
  line L387 (15.367, 24.4488) -> (15.3311, 24.3508)
  line L388 (15.3311, 24.3508) -> (16.0099, 23.9101)
  line L389 (16.0099, 23.9101) -> (16.0848, 23.9827)
  line L390 (16.0848, 23.9827) -> (16.1612, 24.0544)
  line L391 (16.1612, 24.0544) -> (16.3181, 24.1949)
  line L392 (16.3181, 24.1949) -> (16.6465, 24.4656)
  line L393 (16.6465, 24.4656) -> (16.9922, 24.7238)
  line L394 (16.9922, 24.7238) -> (17.3535, 24.9704)
  line L395 (17.3535, 24.9704) -> (17.729, 25.2061)
  line L396 (17.729, 25.2061) -> (18.1179, 25.431)
  line L397 (18.1179, 25.431) -> (18.5876, 25.0898)
  line L398 (18.5876, 25.0898) -> (18.4938, 24.6504)
  line L399 (18.4938, 24.6504) -> (18.3858, 24.2204)
  line L400 (18.3858, 24.2204) -> (18.2628, 23.8006)
  line L401 (18.2628, 23.8006) -> (18.1241, 23.392)
  line L402 (18.1241, 23.392) -> (17.9681, 22.996)
  line L403 (17.9681, 22.996) -> (17.883, 22.8034)
  line L404 (17.883, 22.8034) -> (17.8384, 22.7086)
  line L405 (17.8384, 22.7086) -> (17.7925, 22.6149)
  line L406 (17.7925, 22.6149) -> (18.4214, 22.1056)
  line L407 (18.4214, 22.1056) -> (18.5036, 22.17)
  line L408 (18.5036, 22.17) -> (18.587, 22.2333)
  line L409 (18.587, 22.2333) -> (18.7577, 22.3566)
  line L410 (18.7577, 22.3566) -> (19.1126, 22.5915)
  line L411 (19.1126, 22.5915) -> (19.4834, 22.8122)
  line L412 (19.4834, 22.8122) -> (19.8685, 23.0197)
  line L413 (19.8685, 23.0197) -> (20.2666, 23.2148)
  line L414 (20.2666, 23.2148) -> (20.6769, 23.3979)
  line L415 (20.6769, 23.3979) -> (21.1084, 23.0094)
  line L416 (21.1084, 23.0094) -> (20.9692, 22.5822)
  line L417 (20.9692, 22.5822) -> (20.8168, 22.1659)
  line L418 (20.8168, 22.1659) -> (20.6506, 21.7612)
  line L419 (20.6506, 21.7612) -> (20.4699, 21.3694)
  line L420 (20.4699, 21.3694) -> (20.2734, 20.9919)
  line L421 (20.2734, 20.9919) -> (20.1686, 20.8092)
  line L422 (20.1686, 20.8092) -> (20.1144, 20.7196)
  line L423 (20.1144, 20.7196) -> (20.0589, 20.6312)
  line L424 (20.0589, 20.6312) -> (20.6312, 20.0589)
  line L425 (20.6312, 20.0589) -> (20.7196, 20.1144)
  line L426 (20.7196, 20.1144) -> (20.8092, 20.1686)
  line L427 (20.8092, 20.1686) -> (20.9919, 20.2734)
  line L428 (20.9919, 20.2734) -> (21.3694, 20.4699)
  line L429 (21.3694, 20.4699) -> (21.7612, 20.6506)
  line L430 (21.7612, 20.6506) -> (22.1659, 20.8168)
  line L431 (22.1659, 20.8168) -> (22.5822, 20.9692)
  line L432 (22.5822, 20.9692) -> (23.0094, 21.1084)
  line L433 (23.0094, 21.1084) -> (23.3979, 20.6769)
  line L434 (23.3979, 20.6769) -> (23.2148, 20.2666)
  line L435 (23.2148, 20.2666) -> (23.0197, 19.8685)
  line L436 (23.0197, 19.8685) -> (22.8122, 19.4834)
  line L437 (22.8122, 19.4834) -> (22.5915, 19.1126)
  line L438 (22.5915, 19.1126) -> (22.3566, 18.7577)
  line L439 (22.3566, 18.7577) -> (22.2333, 18.587)
  line L440 (22.2333, 18.587) -> (22.17, 18.5035)
  line L441 (22.17, 18.5035) -> (22.1056, 18.4214)
  line L442 (22.1056, 18.4214) -> (22.6149, 17.7925)
  line L443 (22.6149, 17.7925) -> (22.7086, 17.8384)
  line L444 (22.7086, 17.8384) -> (22.8034, 17.883)
  line L445 (22.8034, 17.883) -> (22.996, 17.9681)
  line L446 (22.996, 17.9681) -> (23.392, 18.1241)
  line L447 (23.392, 18.1241) -> (23.8006, 18.2628)
  line L448 (23.8006, 18.2628) -> (24.2204, 18.3858)
  line L449 (24.2204, 18.3858) -> (24.6504, 18.4938)
  line L450 (24.6504, 18.4938) -> (25.0898, 18.5876)
  line L451 (25.0898, 18.5876) -> (25.431, 18.1179)
  line L452 (25.431, 18.1179) -> (25.2061, 17.729)
  line L453 (25.2061, 17.729) -> (24.9704, 17.3535)
  line L454 (24.9704, 17.3535) -> (24.7238, 16.9922)
  line L455 (24.7238, 16.9922) -> (24.4656, 16.6465)
  line L456 (24.4656, 16.6465) -> (24.1949, 16.3181)
  line L457 (24.1949, 16.3181) -> (24.0544, 16.1612)
  line L458 (24.0544, 16.1612) -> (23.9827, 16.0848)
  line L459 (23.9827, 16.0848) -> (23.91, 16.0099)
  line L460 (23.91, 16.0099) -> (24.3508, 15.3311)
  line L461 (24.3508, 15.3311) -> (24.4488, 15.367)
  line L462 (24.4488, 15.367) -> (24.5478, 15.4014)
  line L463 (24.5478, 15.4014) -> (24.7482, 15.466)
  line L464 (24.7482, 15.466) -> (25.1583, 15.5797)
  line L465 (25.1583, 15.5797) -> (25.5792, 15.675)
  line L466 (25.5792, 15.675) -> (26.0096, 15.7533)
  line L467 (26.0096, 15.7533) -> (26.4485, 15.8158)
  line L468 (26.4485, 15.8158) -> (26.8952, 15.8632)
  line L469 (26.8952, 15.8632) -> (27.1855, 15.3604)
  line L470 (27.1855, 15.3604) -> (26.9212, 14.9971)
  line L471 (26.9212, 14.9971) -> (26.6476, 14.6483)
  line L472 (26.6476, 14.6483) -> (26.3645, 14.3148)
  line L473 (26.3645, 14.3148) -> (26.0716, 13.9979)
  line L474 (26.0716, 13.9979) -> (25.768, 13.6996)
  line L475 (25.768, 13.6996) -> (25.6119, 13.5583)
  line L476 (25.6119, 13.5583) -> (25.5327, 13.4898)
  line L477 (25.5327, 13.4898) -> (25.4526, 13.4229)
  line L478 (25.4526, 13.4229) -> (25.82, 12.7018)
  line L479 (25.82, 12.7018) -> (25.9212, 12.7272)
  line L480 (25.9212, 12.7272) -> (26.0232, 12.7511)
  line L481 (26.0232, 12.7511) -> (26.2293, 12.7943)
  line L482 (26.2293, 12.7943) -> (26.649, 12.8646)
  line L483 (26.649, 12.8646) -> (27.0776, 12.9153)
  line L484 (27.0776, 12.9153) -> (27.5138, 12.9483)
  line L485 (27.5138, 12.9483) -> (27.9568, 12.9646)
  line L486 (27.9568, 12.9646) -> (28.4061, 12.965)
  line L487 (28.4061, 12.965) -> (28.6422, 12.4346)
  line L488 (28.6422, 12.4346) -> (28.3413, 12.1009)
  line L489 (28.3413, 12.1009) -> (28.0328, 11.7826)
  line L490 (28.0328, 11.7826) -> (27.7164, 11.4805)
  line L491 (27.7164, 11.4805) -> (27.3919, 11.196)
  line L492 (27.3919, 11.196) -> (27.0589, 10.9311)
  line L493 (27.0589, 10.9311) -> (26.8888, 10.8068)
  line L494 (26.8888, 10.8068) -> (26.8029, 10.747)
  line L495 (26.8029, 10.747) -> (26.7162, 10.6888)
  line L496 (26.7162, 10.6888) -> (27.0062, 9.9333)
  line L497 (27.0062, 9.9333) -> (27.1095, 9.948)
  line L498 (27.1095, 9.948) -> (27.2135, 9.9611)
  line L499 (27.2135, 9.9611) -> (27.423, 9.9825)
  line L500 (27.423, 9.9825) -> (27.8478, 10.0085)
  line L501 (27.8478, 10.0085) -> (28.2792, 10.0142)
  line L502 (28.2792, 10.0142) -> (28.7165, 10.0014)
  line L503 (28.7165, 10.0014) -> (29.1588, 9.9713)
  line L504 (29.1588, 9.9713) -> (29.6057, 9.9247)
  line L505 (29.6057, 9.9247) -> (29.7851, 9.3725)
  line L506 (29.7851, 9.3725) -> (29.451, 9.0722)
  line L507 (29.451, 9.0722) -> (29.1108, 8.7878)
  line L508 (29.1108, 8.7878) -> (28.7646, 8.5205)
  line L509 (28.7646, 8.5205) -> (28.4122, 8.2715)
  line L510 (28.4122, 8.2715) -> (28.0532, 8.0428)
  line L511 (28.0532, 8.0428) -> (27.8711, 7.937)
  line L512 (27.8711, 7.937) -> (27.7794, 7.8865)
  line L513 (27.7794, 7.8865) -> (27.6871, 7.8377)
  line L514 (27.6871, 7.8377) -> (27.8966, 7.0559)
  line L515 (27.8966, 7.0559) -> (28.0009, 7.0598)
  line L516 (28.0009, 7.0598) -> (28.1056, 7.0619)
  line L517 (28.1056, 7.0619) -> (28.3162, 7.0614)
  line L518 (28.3162, 7.0614) -> (28.7414, 7.0428)
  line L519 (28.7414, 7.0428) -> (29.1711, 7.0034)
  line L520 (29.1711, 7.0034) -> (29.6046, 6.9449)
  line L521 (29.6046, 6.9449) -> (30.0414, 6.8687)
  line L522 (30.0414, 6.8687) -> (30.4809, 6.7757)
  line L523 (30.4809, 6.7757) -> (30.6016, 6.2078)
  line L524 (30.6016, 6.2078) -> (30.2379, 5.944)
  line L525 (30.2379, 5.944) -> (29.8699, 5.6968)
  line L526 (29.8699, 5.6968) -> (29.4976, 5.4671)
  line L527 (29.4976, 5.4671) -> (29.1211, 5.2563)
  line L528 (29.1211, 5.2563) -> (28.7403, 5.0664)
  line L529 (28.7403, 5.0664) -> (28.5481, 4.9802)
  line L530 (28.5481, 4.9802) -> (28.4516, 4.9395)
  line L531 (28.4516, 4.9395) -> (28.3547, 4.9006)
  line L532 (28.3547, 4.9006) -> (28.4813, 4.1013)
  line L533 (28.4813, 4.1013) -> (28.5855, 4.0942)
  line L534 (28.5855, 4.0942) -> (28.6898, 4.0854)
  line L535 (28.6898, 4.0854) -> (28.8992, 4.0628)
  line L536 (28.8992, 4.0628) -> (29.3201, 3.9999)
  line L537 (29.3201, 3.9999) -> (29.7433, 3.9158)
  line L538 (29.7433, 3.9158) -> (30.1684, 3.8123)